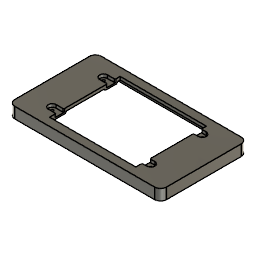
Screen Back (Autodesk Fusion 360 design; units mm, degrees)
Autodesk Fusion 360 part; units mm, degrees
note: some values were not read from the file. Set by a fixed rule: which sketch regions a step uses.
sketch "Sketch1" plane through (0, 0, 0) normal (0, 0, 1) x (1, 0, 0)
  line L0 (-96.825, 55.325) -> (96.825, 55.325)
  line L1 (96.825, 55.325) -> (96.825, -55.325)
  line L2 (96.825, -55.325) -> (-96.825, -55.325)
  line L3 (-96.825, -55.325) -> (-96.825, 55.325)
  line L4 (-86.825, 52.575) -> (86.825, 52.575)
  line L5 (86.825, 52.575) -> (86.825, -52.575)
  line L6 (86.825, -52.575) -> (-86.825, -52.575)
  line L7 (-86.825, -52.575) -> (-86.825, 52.575)
  point P0 (0, 55.325)
  point P1 (96.825, 0)
  point P2 (0, 52.575)
  point P3 (86.825, 0)
  dimension "d1" = 193.65
  dimension "d2" = 110.65
  dimension "d9" = 2.75
  dimension "d10" = 10
  constraint horizontal L0
  constraint vertical L1
  constraint horizontal L2
  constraint vertical L3
  constraint midpoint L0 P0
  constraint midpoint L1 P1
  constraint vertical origin P0
  constraint horizontal origin P1
  constraint horizontal L4
  constraint vertical L5
  constraint horizontal L6
  constraint vertical L7
  constraint midpoint L4 P2
  constraint midpoint L5 P3
  constraint vertical origin P2
  constraint horizontal origin P3
  measures "d1" distance of L0.start L0.end
  measures "d2" distance of L0.end L1.end
  measures "d9" distance of L0 L4
  measures "d10" distance of L1 L5
extrude "Extrude2" add sketch "Sketch1" along normal mid plane 8
fillet "Fillet1" radius 7.5 4 edges at (-96.825, 55.325, 0) (-96.825, -55.325, 0) (96.825, -55.325, 0) (96.825, 55.325, 0)
sketch "Sketch2" plane through (0, 0, 4) normal (0, 0, 1) x (-1, 0, 0)
  arc A0 (-96.825, -47.825) -> (-89.325, -55.325) centre (-89.325, -47.825) ccw
  line L0 (-89.325, -55.325) -> (89.325, -55.325)
  arc A1 (89.325, -55.325) -> (96.825, -47.825) centre (89.325, -47.825) ccw
  line L1 (96.825, -47.825) -> (96.825, 47.825)
  arc A2 (96.825, 47.825) -> (89.325, 55.325) centre (89.325, 47.825) ccw
  line L2 (89.325, 55.325) -> (-89.325, 55.325)
  arc A3 (-89.325, 55.325) -> (-96.825, 47.825) centre (-89.325, 47.825) ccw
  line L3 (-96.825, 47.825) -> (-96.825, -47.825)
  line L4 (-86.825, 52.575) -> (86.825, 52.575)
  line L5 (86.825, 52.575) -> (86.825, -52.575)
  line L6 (86.825, -52.575) -> (-86.825, -52.575)
  line L7 (-86.825, -52.575) -> (-86.825, 52.575)
  line L8 (96.825, -47.825) -> (96.825, 47.825)
  arc A4 (96.825, 47.825) -> (89.325, 55.325) centre (89.325, 47.825) ccw
  line L9 (89.325, 55.325) -> (-89.325, 55.325)
  arc A5 (-89.325, 55.325) -> (-96.825, 47.825) centre (-89.325, 47.825) ccw
  line L10 (-96.825, 47.825) -> (-96.825, -47.825)
  arc A6 (-96.825, -47.825) -> (-89.325, -55.325) centre (-89.325, -47.825) ccw
  line L11 (-89.325, -55.325) -> (89.325, -55.325)
  arc A7 (89.325, -55.325) -> (96.825, -47.825) centre (89.325, -47.825) ccw
  constraint coincident A1.end L1.start
  constraint tangent A1 L8
  constraint coincident A2.end L2.start
  constraint tangent L8 A4
  constraint concentric A2 A4
  constraint coincident L2 A3.start
  constraint coincident A3.end L3.start
  constraint tangent L9 A5
  constraint coincident A0.start L3.end
  constraint coincident A0.end L0.start
  constraint tangent L10 A6
  constraint coincident L0.end A1.start
  constraint tangent L11 A7
  constraint equal A5 A6
extrude "Extrude3" add sketch "Sketch2" along normal blind 6 contours A0 L0 A1 L1 A2 L2 A3 L3 L8 A4 L9 A5 L10 A6 L11 A7 | L4 L5 L6 L7
sketch "Sketch3" plane through (0, 0, 10) normal (0, 0, 1) x (-1, 0, 0)
  arc A0 (89.325, -55.325) -> (96.825, -47.825) centre (89.325, -47.825) ccw
  line L0 (96.825, -47.825) -> (96.825, 47.825)
  arc A1 (96.825, 47.825) -> (89.325, 55.325) centre (89.325, 47.825) ccw
  line L1 (89.325, 55.325) -> (-89.325, 55.325)
  arc A2 (-89.325, 55.325) -> (-96.825, 47.825) centre (-89.325, 47.825) ccw
  line L2 (-96.825, 47.825) -> (-96.825, -47.825)
  arc A3 (-96.825, -47.825) -> (-89.325, -55.325) centre (-89.325, -47.825) ccw
  line L3 (-89.325, -55.325) -> (89.325, -55.325)
  line L4 (72.305, -37.575) -> (-68.825, -37.575) construction
  line L5 (-68.825, -37.575) -> (-68.825, 35.975) construction
  line L6 (-68.825, 35.975) -> (72.305, 35.975) construction
  line L7 (72.305, 35.975) -> (72.305, -37.575) construction
  point P0 (-61.325, -33.575)
  point P1 (-61.325, 31.975)
  point P2 (64.805, -33.575)
  point P3 (64.805, 31.975)
  dimension "d17" = 73.55
  dimension "d18" = 4
  dimension "d19" = 4
  dimension "d20" = 141.13
  dimension "d21" = 7.5
  dimension "d22" = 7.5
  dimension "d23" = 4
  dimension "d24" = 7.5
  dimension "d25" = 4
  dimension "d26" = 7.5
  dimension "d27" = 28
  dimension "d28" = 17.75
  constraint horizontal L4
  constraint vertical L5
  constraint horizontal L6
  constraint vertical L7
  measures "d17" distance of L4.end L5.end
  measures "d18" distance of L4 P0
  measures "d19" distance of L6 P1
  measures "d20" distance of L5.end L6.end
  measures "d21" distance of L5 P0
  measures "d22" distance of L5 P1
  measures "d23" distance of L4 P2
  measures "d24" distance of L7 P2
  measures "d25" distance of L6 P3
  measures "d26" distance of L7 P3
  measures "d27" distance of L2 L5
  measures "d28" distance of L3 L4
extrude "Extrude5" cut 1 faces at (28.9417, -17.525, 4) along direction (0, 0, 1) blind 2
sketch "Sketch4" plane through (0, 0, 10) normal (0, 0, 1) x (-1, 0, 0)
  arc A0 (89.325, -55.325) -> (96.825, -47.825) centre (89.325, -47.825) ccw
  line L0 (96.825, -47.825) -> (96.825, 47.825)
  arc A1 (96.825, 47.825) -> (89.325, 55.325) centre (89.325, 47.825) ccw
  line L1 (89.325, 55.325) -> (-89.325, 55.325)
  arc A2 (-89.325, 55.325) -> (-96.825, 47.825) centre (-89.325, 47.825) ccw
  line L2 (-96.825, 47.825) -> (-96.825, -47.825)
  arc A3 (-96.825, -47.825) -> (-89.325, -55.325) centre (-89.325, -47.825) ccw
  line L3 (-89.325, -55.325) -> (89.325, -55.325)
  line L4 (55, -45) -> (-55, -45)
  line L5 (-55, -45) -> (-55, 45)
  line L6 (-55, 45) -> (55, 45)
  line L7 (55, 45) -> (55, -45)
  point P0 (0, -45)
  dimension "d33" = 110
  dimension "d35" = 45
  dimension "d36" = 45
  constraint horizontal L4
  constraint vertical L5
  constraint horizontal L6
  constraint vertical L7
  constraint midpoint L4 P0
  constraint vertical origin P0
  measures "d33" distance of L5 L7
  measures "d35" distance of origin L4
  measures "d36" distance of origin L6
extrude "Extrude4" cut sketch "Sketch4" against normal through all contours L4 L5 L6 L7
sketch "Sketch5" plane through (0, 0, 6) normal (0, 0, -1) x (1, 0, 0)
  line L0 (86.825, -52.575) -> (86.825, 52.575)
  line L1 (86.825, 52.575) -> (-86.825, 52.575)
  line L2 (-86.825, 52.575) -> (-86.825, -52.575)
  line L3 (-86.825, -52.575) -> (86.825, -52.575)
  circle A0 centre (61.325, -33.575) radius 7.5
  circle A1 centre (61.325, 31.975) radius 7.5
  circle A2 centre (-64.805, -33.575) radius 7.5
  circle A3 centre (-64.805, 31.975) radius 7.5
  line L4 (-55, -45) -> (-55, 45)
  line L5 (-55, 45) -> (55, 45)
  line L6 (55, 45) -> (55, -45)
  line L7 (55, -45) -> (-55, -45)
  line L8 (-64.805, -26.075) -> (-55, -26.075)
  line L9 (-64.805, -41.075) -> (-55, -41.075)
  line L10 (-64.805, 39.475) -> (-55, 39.475)
  line L11 (-64.805, 24.475) -> (-55, 24.475)
  line L12 (61.325, 39.475) -> (55, 39.475)
  line L13 (61.325, 24.475) -> (55, 24.475)
  line L14 (61.325, -26.075) -> (55, -26.075)
  line L15 (61.325, -41.075) -> (55, -41.075)
  point P0 (61.325, -33.575)
  point P1 (-64.805, -33.575)
  point P2 (-64.805, 31.975)
  point P3 (61.325, 31.975)
  dimension "d39" = 15
  dimension "d47" = 126.13
  constraint coincident P0 A0.centre
  constraint coincident P1 A2.centre
  constraint coincident P2 A3.centre
  constraint coincident P3 A1.centre
  constraint equal A0 A1
  constraint equal A1 A3
  constraint equal A2 A3
  constraint coincident A2 L8.start
  constraint coincident L4 L8.end
  constraint tangent A2 L8
  constraint perpendicular L4 L8
  constraint coincident A2 L9.start
  constraint coincident L4 L9.end
  constraint tangent A2 L9
  constraint perpendicular L4 L9
  constraint coincident A3 L10.start
  constraint coincident L4 L10.end
  constraint perpendicular L4 L10
  constraint coincident A3 L11.start
  constraint coincident L4 L11.end
  constraint tangent A3 L11
  constraint perpendicular L4 L11
  constraint coincident A1 L12.start
  constraint coincident L6 L12.end
  constraint tangent A1 L12
  constraint coincident A1 L13.start
  constraint coincident L6 L13.end
  constraint tangent A1 L13
  constraint perpendicular L6 L13
  constraint coincident A0 L14.start
  constraint coincident L6 L14.end
  constraint tangent A0 L14
  constraint perpendicular L6 L14
  constraint coincident A0 L15.start
  constraint coincident L6 L15.end
  constraint tangent A0 L15
  constraint perpendicular L6 L15
  constraint horizontal L12
  constraint tangent A3 L10
  measures "d39" diameter of A0
  measures "d47" distance of P0 P1
extrude "Extrude6" add sketch "Sketch5" along normal blind 2 contours A0 L6 | A0 L6 L14 | A0 L6 L15 | A1 L6 L13 | A1 L6 | A1 L6 L12 | A2 L4 L8 L9 | A2 | A3 L4 L10 L11 | A3 picked at (59.7964, -33.5066) picked at (59.5829, 32.3308)
sketch "Sketch6" plane through (0, 0, 10) normal (0, 0, 1) x (-1, 0, 0)
  line L0 (55, 45) -> (55, -45)
  line L1 (55, -45) -> (-55, -45)
  line L2 (-55, -45) -> (-55, 45)
  line L3 (-55, 45) -> (55, 45)
  arc A0 (89.325, -55.325) -> (96.825, -47.825) centre (89.325, -47.825) ccw
  line L4 (96.825, -47.825) -> (96.825, 47.825)
  arc A1 (96.825, 47.825) -> (89.325, 55.325) centre (89.325, 47.825) ccw
  line L5 (89.325, 55.325) -> (-89.325, 55.325)
  arc A2 (-89.325, 55.325) -> (-96.825, 47.825) centre (-89.325, 47.825) ccw
  line L6 (-96.825, 47.825) -> (-96.825, -47.825)
  arc A3 (-96.825, -47.825) -> (-89.325, -55.325) centre (-89.325, -47.825) ccw
  line L7 (-89.325, -55.325) -> (89.325, -55.325)
  circle A4 centre (64.805, -33.575) radius 5
  circle A5 centre (64.805, 31.975) radius 5
  circle A6 centre (-61.325, -33.575) radius 5
  circle A7 centre (-61.325, 31.975) radius 5
  line L8 (64.805, -38.575) -> (55, -38.575)
  line L9 (64.805, -28.575) -> (55, -28.575)
  line L10 (64.805, 26.975) -> (55, 26.975)
  line L11 (64.805, 36.975) -> (55, 36.975)
  line L12 (-61.325, 36.975) -> (-55, 36.975)
  line L13 (-61.325, 26.975) -> (-55, 26.975)
  line L14 (-61.325, -28.575) -> (-55, -28.575)
  line L15 (-61.325, -38.575) -> (-55, -38.575)
  point P0 (64.805, -33.575)
  point P1 (64.805, 31.975)
  point P2 (-61.325, 31.975)
  point P3 (-61.325, -33.575)
  dimension "d44" = 10
  constraint coincident P0 A4.centre
  constraint coincident P1 A5.centre
  constraint coincident P2 A7.centre
  constraint coincident P3 A6.centre
  constraint equal A4 A6
  constraint equal A4 A7
  constraint equal A4 A5
  constraint coincident A4 L8.start
  constraint coincident L0 L8.end
  constraint perpendicular L0 L8
  constraint coincident A4 L9.start
  constraint coincident L0 L9.end
  constraint perpendicular L0 L9
  constraint coincident A5 L10.start
  constraint coincident L0 L10.end
  constraint tangent A5 L10
  constraint coincident A5 L11.start
  constraint coincident L0 L11.end
  constraint tangent A5 L11
  constraint coincident A7 L12.start
  constraint coincident L2 L12.end
  constraint coincident A7 L13.start
  constraint coincident L2 L13.end
  constraint tangent A7 L13
  constraint parallel L11 L13
  constraint coincident A6 L14.start
  constraint coincident L2 L14.end
  constraint tangent A6 L14
  constraint coincident A6 L15.start
  constraint coincident L2 L15.end
  constraint tangent A6 L15
  constraint tangent A4 L8
  constraint tangent A4 L9
  constraint tangent A7 L12
  constraint horizontal L15
  constraint horizontal L14
  constraint horizontal L13
  constraint horizontal L12
  constraint horizontal L10
  measures "d44" diameter of A4
extrude "Extrude7" cut sketch "Sketch6" against normal blind 4 contours L0 A5 L10 L11 | A5 | L2 A7 L12 L13 | L0 A4 L8 L9 | A7 | A4 | L2 A6 L14 L15 | A6
hole "Hole1" at (-64.805, 33.575, 10) at (61.325, 33.575, 10) at (61.325, -31.975, 10) at (-64.805, -31.975, 10) direction (0, 0, -1) diameter 3.4 end through all counterbore diameter 6.5 counterbore depth 3
fillet "Fillet3" radius 1 8 edges at (-55, 28.575, 8) (-55, 38.575, 8) (55, 38.575, 8) (55, 28.575, 8) (55, -26.975, 8) (55, -36.975, 8) (-55, -26.975, 8) (-55, -36.975, 8)
fillet "Fillet4" radius 2 12 edges at (-59.9025, -24.475, 6) (-72.305, -31.975, 6) (-59.9025, -39.475, 6) (-59.9025, 41.075, 6) (-72.305, 33.575, 6) (-59.9025, 26.075, 6) (58.1625, 26.075, 6) (68.825, 33.575, 6) (58.1625, 41.075, 6) (58.1625, -39.475, 6) (68.825, -31.975, 6) (58.1625, -24.475, 6)
equation "d1 = 193.75 mm - 0.1 mm"
equation "d2 = 110.75 mm - 0.1 mm"
equation "d9 = 2.00 mm + 0.75 mm"
equation "d11 = 6 mm + 2 mm"
equation "d19 = d18"
equation "d22 = d21"
equation "d23 = d18"
equation "d24 = d21"
equation "d25 = d23"
equation "d26 = d24"
